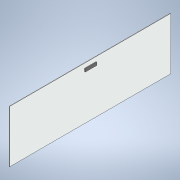
# Autodesk Inventor part: acrilicoMovel1
Saved by Autodesk Inventor 2022 (Build 260153000, 153)
## iProperties
Created: 2022-08-29
Part Number: acrilicoMovel1
Material: Generic
Document SubType Name: Modeling
Designer: cvss2
Density: 1 g/cm^3
Appearance: Default
Author: cvss2
Autodesk Inventor part; units mm, degrees
ref_plane "YZ Plane" through (0, 0, 0) normal (1, 0, 0) x (0, 1, 0)
ref_plane "XZ Plane" through (0, 0, 0) normal (0, 1, 0) x (-1, 0, 0)
ref_plane "XY Plane" through (0, 0, 0) normal (0, 0, 1) x (1, 0, 0)
sketch "Sketch1" plane through (0, 0, 0) normal (1, 0, 0) x (0, 1, 0)
  line L0 (0, 0) -> (-363, 0)
  line L1 (-363, 0) -> (-363, 1118)
  line L2 (-363, 1118) -> (0, 1118)
  line L3 (0, 1118) -> (0, 0)
  dimension "d0" = 363
  dimension "d1" = 1118
  constraints: 8 end point, 2 parallel, 1 horizontal, 1 perpendicular
  measures "d0" distance of L1.end L2.end
  measures "d1" distance of L0.end L1.end
extrude "Extrusion1" add sketch "Sketch1" against normal blind 3
sketch "Sketch2" plane through (0, 0, 0) normal (1, 0, 0) x (0, 0, -1)
  line L0 (-1118, 0) -> (-1118, -363) projected
  line L1 (-1118, -363) -> (0, -363) projected
  line L2 (0, -363) -> (0, 0) projected
  line L3 (0, 0) -> (-1118, 0) projected
  line L4 (-1118, 0) -> (0, 0) construction
  line L5 (-559, 0) -> (-559, -40) construction
  line L6 (-519, -30) -> (-599, -30)
  line L7 (-599, -30) -> (-599, -50)
  line L8 (-599, -50) -> (-519, -50)
  line L9 (-519, -50) -> (-519, -30)
  line L10 (-519, -30) -> (-599, -50) construction
  line L11 (-599, -30) -> (-519, -50) construction
  dimension "d4" = 40
  dimension "d5" = 80
  dimension "d6" = 20
  constraints: 14 end point, 3 midpoint, 2 parallel, 1 horizontal, 1 perpendicular, 1 vertical
  measures "d4" distance of L5.start L5.end
  measures "d5" distance of L8.end L7.end
  measures "d6" distance of L7.end L6.end
extrude "Extrusion2" add sketch "Sketch2" along normal blind 6 and the other way blind 9 contours L9 L8 L7 L6
equation "\"d0\" = portaLargura"
equation "\"portaLargura\" = 363"
body "Solid1"
